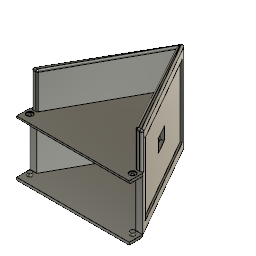
RoofWireBoxAirQualityHoboken v4 (Autodesk Fusion 360 design; units mm, degrees)
Autodesk Fusion 360 part; units mm, degrees
sketch "Sketch1" plane through (0, 0, 0) normal (0, 0, 1) x (1, 0, 0)
  line L0 (0, 0) -> (62.725, 0)
  line L1 (0, 0) -> (-62.725, 0)
  line L2 (62.725, 0) -> (62.725, -15)
  circle A0 centre (-57.125, -5.6) radius 1.5
  line L3 (-62.725, 0) -> (-62.725, -15)
  line L4 (-62.725, -15) -> (62.725, -15)
  circle A1 centre (57.125, -5.6) radius 1.5
  line L5 (0, 0) -> (0, 109.7609) construction
  line L6 (-62.725, 0) -> (0, 109.7609)
  line L7 (62.725, 0) -> (0, 109.7609)
  line L8 (0, 109.7609) -> (0, 100)
  line L9 (0, 100) -> (-55, 0)
  line L10 (0, 100) -> (55, 0)
  circle A2 centre (-57.125, -5.6) radius 3.5
  circle A3 centre (57.125, -5.6) radius 3.5
  dimension "d1" = 62.725
  dimension "d2" = 62.725
  dimension "d3" = 15
  dimension "d8" = 3
  dimension "d9" = 15
  dimension "d12" = 3
  dimension "d33" = 2
  dimension "d34" = 2
  constraint coincident L0.start L1.start
  constraint horizontal L0
  constraint parallel L0 L1
  constraint perpendicular L0 L2
  constraint perpendicular L1 L3
  constraint perpendicular L0 L5
  constraint coincident L5 L8.end
  constraint coincident L1 L9.end
  constraint coincident L0 L10.end
  measures "d1" distance of L0.start L0.end
  measures "d2" distance of L0.start L1.end
  measures "d3" distance of L0.end L2.end
  measures "d8" diameter of A0
  measures "d9" distance of L1.end L3.end
  measures "d12" diameter of A1
extrude "Extrude1" add sketch "Sketch1" against normal blind 3 contours L0 L1 L2 L3 L4 | A2 | A3 makes body 1
extrude "Extrude2" add sketch "Sketch1" against normal blind 62 separate body contours L0 L7 L8 L10 | L1 L6 L8 L9 makes body 2
extrude "Extrude3" add sketch "Sketch1" against normal blind 3 contours L0 L1 L9 L10 bodies 1 2
sketch "Sketch2" plane through (0, 0, -62) normal (0, 0, -1) x (1, 0, 0)
  line L0 (0, -100) -> (-55, 0)
  line L1 (-55, 0) -> (-62.725, 0)
  line L2 (-62.725, 0) -> (0, -109.7609)
  line L3 (0, -109.7609) -> (62.725, 0)
  line L4 (55, 0) -> (0, -100)
  line L5 (0, 0) -> (-62.725, 0)
  line L6 (0, 0) -> (62.725, 0)
  line L7 (62.725, 0) -> (62.725, 15)
  line L8 (-62.725, 0) -> (-62.725, 15)
  line L9 (-62.725, 15) -> (62.725, 15)
  line L10 (62.725, 0) -> (55, 0)
  circle A0 centre (57.125, 5.6) radius 2.5
  circle A1 centre (-57.125, 5.6) radius 2.5
  dimension "d23" = 5
  dimension "d24" = 5.6
  dimension "d25" = 5.6
  dimension "d26" = 5
  dimension "d27" = 5.6
  dimension "d28" = 5.6
  constraint coincident L5.start L6.start
  constraint coincident L1.end L2.start
  constraint coincident L3.end L6.end
  constraint perpendicular L6 L7
  constraint perpendicular L1 L8
  constraint perpendicular L7 L9
  measures "d23" diameter of A0
  measures "d24" distance of L6 A0.centre
  measures "d25" distance of L7 A0.centre
  measures "d26" diameter of A1
  measures "d27" distance of L5 A1.centre
  measures "d28" distance of L8 A1.centre
extrude "Extrude4" add sketch "Sketch2" against normal blind 3 separate body contours L1 L5 L6 L7 L8 L9 L10 | A0 | A1 makes body 3
extrude "Extrude5" add sketch "Sketch2" against normal blind 3 contours L0 L4 L5 L6 bodies 1 3
extrude "Extrude6" add sketch "Sketch2" against normal blind 6 contours A0 | A1 bodies 1
extrude "Extrude7" cut sketch "Sketch1" against normal blind 1 contours A2 | A3 bodies 1
chamfer "Chamfer1" distance 1 angle 45 1 edges at (0, -15, -3) on bodies 1
extrude "Extrude8" add sketch "Sketch1" along normal blind 40 contours L0 L7 L8 L10 | L1 L6 L8 L9 bodies 1
sketch "Sketch3" plane through (-47.2833, 27.021, 0) normal (-0.868228, 0.496166, 0) x (-0.496166, -0.868228, 0)
  line L0 (-95.2975, 40) -> (-95.2975, -62)
  line L1 (-95.2975, -62) -> (31.122, -62)
  line L2 (31.122, -62) -> (31.122, -59)
  line L3 (31.122, -59) -> (31.122, -3)
  line L4 (31.122, -3) -> (31.122, 0)
  line L5 (31.122, 0) -> (31.122, 40)
  line L6 (31.122, 40) -> (-95.2975, 40)
  line L7 (-87.0975, 29) -> (22.9025, 29) construction
  line L8 (22.9025, 29) -> (22.9025, -51) construction
  line L9 (22.9025, -51) -> (-87.0975, -51) construction
  line L10 (-87.0975, -51) -> (-87.0975, 29) construction
  line L11 (23.5025, -51.6) -> (-87.6975, -51.6) construction
  line L12 (-87.6975, -51.6) -> (-87.6975, 29.6) construction
  line L13 (-87.6975, 29.6) -> (23.5025, 29.6) construction
  line L14 (23.5025, 29.6) -> (23.5025, -51.6) construction
  line L15 (-54.0975, -4) -> (-10.0975, -4)
  line L16 (-10.0975, -4) -> (-10.0975, -18)
  line L17 (-10.0975, -18) -> (-54.0975, -18)
  line L18 (-54.0975, -18) -> (-54.0975, -4)
  line L19 (-87.2975, 29.2) -> (23.1025, 29.2)
  line L20 (23.1025, 29.2) -> (23.1025, -51.2)
  line L21 (23.1025, -51.2) -> (-87.2975, -51.2)
  line L22 (-87.2975, -51.2) -> (-87.2975, 29.2)
  line L23 (-41.0975, -4) -> (-41.0975, -18)
  line L24 (-23.0975, -4) -> (-23.0975, -18)
  line L25 (-23.0975, -18) -> (-41.0975, -18)
  line L26 (-23.0975, -4) -> (-41.0975, -4)
  dimension "d40" = 110
  dimension "d41" = 80
  dimension "d42" = 11
  dimension "d43" = 8.2
  dimension "d44" = -0.6
  dimension "d55" = 33
  dimension "d66" = -0.2
  dimension "d67" = 13
  dimension "d68" = 13
  constraint horizontal L7
  constraint vertical L8
  constraint horizontal L9
  constraint vertical L10
  constraint coincident L15 L23.start
  constraint coincident L17 L23.end
  constraint perpendicular L17 L23
  constraint coincident L15 L24.start
  constraint coincident L17 L24.end
  constraint perpendicular L17 L24
  measures "d40" distance of L7.start L7.end
  measures "d41" distance of L7.start L9.end
  measures "d42" distance of L6 L7
  measures "d43" distance of L0 L10
  measures "d67" distance of L18 L23
  measures "d68" distance of L16 L24
extrude "Extrude12" cut sketch "Sketch3" against normal blind 2 contours L15 L17 L18 L23 | L15 L17 L23 L24 L25 L26 | L15 L16 L17 L24 | L19 L20 L21 L22 bodies 1
extrude "Extrude13" cut sketch "Sketch3" against normal blind 15 contours L15 L17 L23 L24 L25 L26 bodies 1
mirror "Mirror2" about plane through (0, 0, 0) normal (1, 0, 0) of "Extrude12", "Extrude13"
fillet "Fillet2" radius 2 5 edges at (31.3625, 54.8805, 40) (-31.3625, 54.8805, 40) (0, 109.7609, -11) (31.3625, 54.8805, -62) (-31.3625, 54.8805, -62) on bodies 1
fillet "Fillet2" radius 2 8 edges at (-27.5, 50, 40) (27.5, 50, 40) (-55, 0, 20) (-62.725, 0, 20) (55, 0, 20) (62.725, 0, 20) (-58.8625, 0, 40) (58.8625, 0, 40) on bodies 1
equation "d15 = -56 mm - 6 mm"
